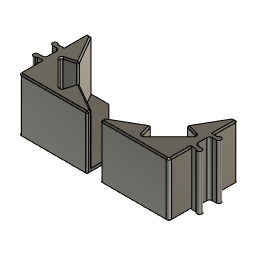
LED_strip_mount (Autodesk Fusion 360 design; units mm, degrees)
Autodesk Fusion 360 part; units mm, degrees
sketch "Sketch1" plane through (0, 0, 0) normal (0, 0, 1) x (1, 0, 0)
  line L0 (0, 0) -> (0, 19.6)
  line L1 (2.6196, 10.3253) -> (5.7353, 11.2005)
  line L2 (5.9735, 11.7856) -> (1.3464, 19.8)
  line L3 (1, 20) -> (0.4, 20)
  line L4 (0, 0) -> (6.0511, 6.0511) construction
  line L5 (2.4449, 9.6574) -> (6.0511, 6.0511)
  arc A0 (2.6196, 10.3253) -> (2.4449, 9.6574) centre (2.7277, 9.9402) ccw
  arc A1 (5.7353, 11.2005) -> (5.9735, 11.7856) centre (5.6271, 11.5856) ccw
  arc A2 (1.3464, 19.8) -> (1, 20) centre (1, 19.6) ccw
  arc A3 (0.4, 20) -> (0, 19.6) centre (0.4, 19.6) ccw
  line L6 (0, 0) -> (19.6, 0)
  line L7 (9.6574, 2.4449) -> (6.0511, 6.0511)
  arc A4 (9.6574, 2.4449) -> (10.3253, 2.6196) centre (9.9402, 2.7277) ccw
  line L8 (10.3253, 2.6196) -> (11.2005, 5.7353)
  arc A5 (11.7856, 5.9735) -> (11.2005, 5.7353) centre (11.5856, 5.6271) ccw
  line L9 (11.7856, 5.9735) -> (19.8, 1.3464)
  arc A6 (20, 1) -> (19.8, 1.3464) centre (19.6, 1) ccw
  line L10 (20, 1) -> (20, 0.4)
  arc A7 (19.6, 0) -> (20, 0.4) centre (19.6, 0.4) ccw
  point P0 (0, 20)
  point P1 (6.2309, 11.3397)
  point P2 (1.2309, 20)
  dimension "d1" = 20
  dimension "d4" = 135
  dimension "d5" = 10
  dimension "d7" = 0.4
  dimension "d8" = 0.4
  dimension "d9" = 0.4
  dimension "d10" = 0.6
  dimension "d11" = 5.1
  dimension "d12" = 4
  dimension "d13" = 30
  constraint coincident L0.start L4.start
  constraint vertical L0
  constraint perpendicular L0 L3
  constraint coincident L4.end L5.end
  constraint perpendicular L4 L5
  constraint tangent L1 A0
  constraint tangent L5 A0
  constraint coincident P1 L1
  constraint coincident P1 L2
  constraint tangent L1 A1
  constraint tangent L2 A1
  constraint coincident P2 L2
  constraint coincident P2 L3
  constraint tangent L2 A2
  constraint tangent L3 A2
  constraint coincident P0 L0
  constraint coincident P0 L3
  constraint tangent L0 A3
  constraint tangent L3 A3
  constraint equal A2 A3
  constraint symmetric L0.start L4 L6.start
  constraint symmetric L4 L5.end L7.end
  constraint symmetric L4 L1.start A4.end
  constraint symmetric L4 L5.start L7.start
  constraint symmetric L4 A0 A4
  constraint symmetric L4 L1.end L8.end
  constraint symmetric L4 L2.start A5.start
  constraint symmetric L4 A1 A5
  constraint symmetric L4 L2.end L9.end
  constraint symmetric L4 L3.start A6.start
  constraint symmetric L4 A2 A6
  constraint symmetric L4 L0.end L6.end
  constraint symmetric L4 L3.end L10.end
  constraint symmetric L4 A3 A7
  measures "d1" distance of L0.start P0
  measures "d4" angle of L0 L4
  measures "d5" distance of P1 P2
  measures "d7" radius of A0
  measures "d8" radius of A1
  measures "d9" radius of A2
  measures "d10" distance of A2.centre A3.centre
  measures "d11" distance of L4.end L5.start
  measures "d12" distance of L5 L2.start
  measures "d13" angle of L0 L2
extrude "Extrude1" add sketch "Sketch1" along normal blind 16 makes body 1
sketch "Sketch2" plane through (0, 0, 0) normal (0, 0, -1) x (1, 0, 0)
  line L0 (19.6, 0) -> (0, 0)
  line L1 (0, 0) -> (0, -19.6)
  arc A0 (0, -19.6) -> (0.4, -20) centre (0.4, -19.6) ccw
  line L2 (0.4, -20) -> (1, -20)
  arc A1 (1, -20) -> (1.3464, -19.8) centre (1, -19.6) ccw
  line L3 (1.3464, -19.8) -> (5.9735, -11.7856)
  arc A2 (5.9735, -11.7856) -> (5.7353, -11.2005) centre (5.6271, -11.5856) ccw
  line L4 (5.7353, -11.2005) -> (2.6196, -10.3253)
  arc A3 (2.4449, -9.6574) -> (2.6196, -10.3253) centre (2.7277, -9.9402) ccw
  line L5 (2.4449, -9.6574) -> (9.6574, -2.4449)
  arc A4 (10.3253, -2.6196) -> (9.6574, -2.4449) centre (9.9402, -2.7277) ccw
  line L6 (10.3253, -2.6196) -> (11.2005, -5.7353)
  arc A5 (11.2005, -5.7353) -> (11.7856, -5.9735) centre (11.5856, -5.6271) ccw
  line L7 (11.7856, -5.9735) -> (19.8, -1.3464)
  arc A6 (19.8, -1.3464) -> (20, -1) centre (19.6, -1) ccw
  line L8 (20, -1) -> (20, -0.4)
  arc A7 (20, -0.4) -> (19.6, 0) centre (19.6, -0.4) ccw
  line L9 (1, -20) -> (6, -20)
  line L10 (6.7071, -19.7071) -> (13.2071, -13.2071)
  line L11 (13.2071, -13.2071) -> (0, 0) construction
  arc A8 (6, -20) -> (6.7071, -19.7071) centre (6, -19) ccw
  line L12 (5.7353, -11.2005) -> (6.0055, -11.2764)
  line L13 (6.3965, -11.1742) -> (8.7853, -8.7853)
  line L14 (5.9735, -11.7856) -> (6.2309, -11.3397) construction
  arc A9 (6.0055, -11.2764) -> (6.3965, -11.1742) centre (6.1137, -10.8913) ccw
  line L15 (11.1742, -6.3965) -> (8.7853, -8.7853)
  line L16 (11.2005, -5.7353) -> (11.2764, -6.0055)
  arc A10 (11.1742, -6.3965) -> (11.2764, -6.0055) centre (10.8913, -6.1137) ccw
  line L17 (19.7071, -6.7071) -> (13.2071, -13.2071)
  arc A11 (19.7071, -6.7071) -> (20, -6) centre (19, -6) ccw
  line L18 (20, -1) -> (20, -6)
  dimension "d16" = 45
  dimension "d17" = 1
  dimension "d18" = 6
  dimension "d19" = 0.4
  constraint coincident L2.end A1.start
  constraint tangent A1 L9
  constraint coincident L0.end L1.start
  constraint tangent L9 A8
  constraint tangent L10 A8
  constraint perpendicular L10 L11
  constraint coincident A2.end L4.start
  constraint tangent A2 L12
  constraint coincident L11 L13.end
  constraint perpendicular L11 L13
  constraint coincident L3.end A2.start
  constraint tangent A2 L14
  constraint coincident L14.end L12
  constraint coincident L14.end L13
  constraint tangent L12 A9
  constraint tangent L13 A9
  constraint symmetric L2.end L11 A6.end
  constraint symmetric L10.end L11 L17.end
  constraint symmetric L11 L9.end A11.end
  constraint symmetric L11 L10.start L17.start
  constraint symmetric L11 A8 A11
  constraint symmetric L11 A2.end L6.end
  constraint symmetric L11 L13.end L15.end
  constraint symmetric L11 L12.end L16.end
  constraint symmetric L11 L13.start L15.start
  constraint symmetric L11 A9 A10
  measures "d16" angle of L0 L11
  measures "d17" radius of A8
  measures "d18" distance of L1 L9.end
  measures "d19" radius of A9
extrude "Extrude2" add sketch "Sketch2" against normal blind 1.2 contours A1 L3 A2 A5 L7 A6 L9 L10 A8 L12 L13 A9 L15 L16 A10 L17 A11 L18 bodies 1
sketch "Sketch3" plane through (0, 0, 16) normal (0, 0, 1) x (-1, 0, 0)
  line L0 (0, 0) -> (-19.6, 0)
  arc A0 (-19.6, 0) -> (-20, -0.4) centre (-19.6, -0.4) ccw
  line L1 (-20, -0.4) -> (-20, -1)
  arc A1 (-20, -1) -> (-19.8, -1.3464) centre (-19.6, -1) ccw
  line L2 (-19.8, -1.3464) -> (-11.7856, -5.9735)
  arc A2 (-11.7856, -5.9735) -> (-11.2005, -5.7353) centre (-11.5856, -5.6271) ccw
  line L3 (-11.2005, -5.7353) -> (-10.3253, -2.6196)
  arc A3 (-9.6574, -2.4449) -> (-10.3253, -2.6196) centre (-9.9402, -2.7277) ccw
  line L4 (-9.6574, -2.4449) -> (-2.4449, -9.6574)
  arc A4 (-2.6196, -10.3253) -> (-2.4449, -9.6574) centre (-2.7277, -9.9402) ccw
  line L5 (-2.6196, -10.3253) -> (-5.7353, -11.2005)
  arc A5 (-5.7353, -11.2005) -> (-5.9735, -11.7856) centre (-5.6271, -11.5856) ccw
  line L6 (-5.9735, -11.7856) -> (-1.3464, -19.8)
  arc A6 (-1.3464, -19.8) -> (-1, -20) centre (-1, -19.6) ccw
  line L7 (-1, -20) -> (-0.4, -20)
  arc A7 (-0.4, -20) -> (0, -19.6) centre (-0.4, -19.6) ccw
  line L8 (0, -19.6) -> (0, 0)
  line L9 (0, -9.8) -> (-2.3531, -9.8) construction
  line L10 (0, -7.7) -> (2, -7.7)
  arc A8 (2, -7.7) -> (1.597, -6.422) centre (2, -6.9975) ccw
  line L11 (1.597, -6.422) -> (1.2, -6.7)
  line L12 (1.2, -6.7) -> (0, -6.7)
  line L13 (1.2, -12.9) -> (0, -12.9)
  line L14 (1.597, -13.178) -> (1.2, -12.9)
  arc A9 (1.597, -13.178) -> (2, -11.9) centre (2, -12.6025) ccw
  line L15 (0, -11.9) -> (2, -11.9)
  dimension "d22" = 1
  dimension "d23" = 145
  dimension "d24" = 1.2
  dimension "d25" = 2
  dimension "d26" = 3.1
  constraint midpoint L8 L9.start
  constraint coincident A4 L9.end
  constraint perpendicular L8 L9
  constraint coincident L8 L10.start
  constraint perpendicular L8 L10
  constraint tangent A8 L11
  constraint coincident L8 L12.end
  constraint perpendicular L8 L12
  constraint tangent L10 A8
  constraint symmetric L9 L10.start L15.start
  constraint symmetric L9 L10.end A9.end
  constraint symmetric L9 A8.end L14.start
  constraint symmetric L9 A8 A9
  constraint symmetric L9 L11.end L13.start
  constraint symmetric L9 L12.end L13.end
  measures "d22" distance of L10 L12
  measures "d23" angle of L11 L12
  measures "d24" distance of L11.end L12.end
  measures "d25" distance of L10.start L10.end
  measures "d26" distance of L9 L12
extrude "Extrude3" add sketch "Sketch3" against normal up to surface (16 mm away) contours L8 L10 A8 L11 L12 | L8 L13 L14 A9 L15 bodies 1
fillet "Fillet1" radius 0.8 3 edges at (0, 11.9, 8) (0, 7.7, 8) (0, 0, 8) on bodies 1
chamfer "Chamfer1" distance 0.4 angle 45 38 edges at (0, 16.25, 16) (0, 3.75, 16) (0.2343, 0.2343, 16) (10.2, 0, 16) (19.8828, 0.1172, 16) (20, 0.7, 16) (19.9464, 1.2, 16) (15.7928, 3.66, 16) (11.4348, 5.9976, 16) (10.7629, 4.1774, 16) (10.0414, 2.3408, 16) (6.0511, 6.0511, 16) (2.3408, 10.0414, 16) (4.1774, 10.7629, 16) (5.9976, 11.4348, 16) (3.66, 15.7928, 16) (1.2, 19.9464, 16) (0.7, 20, 16) (0.1172, 19.8828, 16) (0, 3.75, 0) (0, 16.25, 0) (0.1172, 19.8828, 0) (3.2, 20, 0) (6.3827, 19.9239, 0) (13.2071, 13.2071, 0) (19.9239, 6.3827, 0) (20, 3.2, 0) (19.8828, 0.1172, 0) (10.2, 0, 0) (0.2343, 0.2343, 0) (8.7853, 8.7853, 0) (6.2149, 11.2783, 0) (4.3125, 10.8009, 0) (2.3408, 10.0414, 0) (6.0511, 6.0511, 0) (10.0414, 2.3408, 0) (10.8009, 4.3125, 0) (11.2783, 6.2149, 0) on bodies 1
ref_plane "WorkPlane1" through (22, 0, 0) normal (1, 0, 0) x (0, 1, 0)
mirror "Mirror1" about plane through (22, 0, 0) normal (1, 0, 0) of bodies 1 makes body 2
equation "d8 = d7"
equation "d9 = d7"
equation "d11 = ( 11 / 2 ) * 1 mm - 0.4 mm"
equation "d26 = ( 6.2 / 2 ) * 1 mm"
named bodies: "LED_strip_mount", "LED_strip_mount (mirror)"
